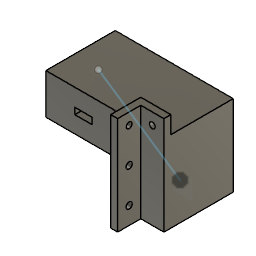
motor_support_strud_Right_v1 (Autodesk Fusion 360 design; units mm, degrees)
part number: 2025-12-05-13-27-42-800
Autodesk Fusion 360 part; units mm, degrees
note: some values were not read from the file. Set by a fixed rule: which sketch regions a step uses.
sketch "Sketch3" plane through (0, 0, 0) normal (0, 0, 1) x (1, 0, 0)
  line L0 (0, 0) -> (-40, 0)
  line L1 (-40, 0) -> (-40, 60)
  line L2 (-40, 60) -> (0, 60)
  line L3 (0, 60) -> (0, 0)
  line L4 (-17.9857, 0) -> (-23.9857, 0)
  line L5 (-23.9857, 0) -> (-23.9857, -20)
  line L6 (-23.9857, -20) -> (-17.9857, -20)
  line L7 (-17.9857, -20) -> (-17.9857, 0)
  line L8 (-40, 0) -> (-23.9857, -20)
  line L9 (-17.9857, 0) -> (2.0143, 0)
  line L10 (2.0143, 0) -> (2.0143, 1.9843)
  line L11 (2.0143, 1.9843) -> (2.0143, 60)
  line L12 (2.0143, 60) -> (0, 60)
  dimension "d16" = 60
  dimension "d17" = 40
  dimension "d18" = 20
  dimension "d19" = 6
  dimension "d63" = 20
  constraint horizontal L0
  constraint vertical L1
  constraint horizontal L2
  constraint vertical L3
  constraint coincident L0.start L3.end
  constraint horizontal L4
  constraint vertical L5
  constraint horizontal L6
  constraint vertical L7
  constraint coincident L0 L4.start
  constraint perpendicular L3 L9
  constraint perpendicular L9 L10
  constraint perpendicular L9 L11
  constraint perpendicular L3 L12
  measures "d16" distance of L0.start L2.end
  measures "d17" distance of L0.start L0.end
  measures "d18" distance of L4.end L5.end
  measures "d19" distance of L5.end L6.end
  measures "d63" distance of L4.start L9.end
extrude "Extrude1" add sketch "Sketch3" along normal blind 85 contours L0 L1 L2 L3 L4 L9 | L0 L4 L5 L6 L7 | L0 L5 L8
sketch "Sketch5" plane through (0, 0, 85) normal (0, 0, 1) x (-1, 0, 0)
  line L0 (23.9857, 20) -> (17.9857, 20)
  line L1 (17.9857, 20) -> (17.9857, 0)
  line L2 (17.9857, 0) -> (0, 0)
  line L3 (0, 0) -> (0, -60)
  line L4 (0, -60) -> (40, -60)
  line L5 (40, -60) -> (40, 0)
  line L6 (40, -60) -> (0, -60)
  line L7 (0, -6) -> (23.9857, -6)
  line L8 (23.9857, -6) -> (23.9857, 0)
  line L9 (40, 0) -> (23.9857, 20)
  line L10 (23.9857, 0) -> (23.9857, 20)
  dimension "d20" = 6
  constraint coincident L4.end L5.start
  constraint coincident L3.end L4.start
  constraint coincident L3 L7.start
  constraint perpendicular L3 L7
  constraint perpendicular L7 L8
  constraint coincident L0.start L9.end
  constraint perpendicular L0 L10
  measures "d20" distance of L2 L7
extrude "Extrude2" cut sketch "Sketch5" against normal blind 15 contours L3 L4 L5 L6 L7 L8 L9 L10
sketch "Sketch6" plane through (-40, 0, 0) normal (-1, 0, 0) x (0, -1, 0)
  line L0 (0, 70) -> (-60, 70)
  line L1 (-60, 70) -> (-60, 0)
  line L2 (-60, 0) -> (0, 0)
  line L3 (-55, 0) -> (-10, 0)
  line L4 (-10, 0) -> (-10, 60)
  line L5 (-10, 60) -> (-55, 60)
  line L6 (-55, 60) -> (-55, 0)
  line L7 (0, 0) -> (0, 70)
  dimension "d23" = 45
  dimension "d27" = 10
  dimension "d28" = 60
  constraint horizontal L3
  constraint vertical L4
  constraint horizontal L5
  constraint vertical L6
  constraint coincident L2 L3.start
  measures "d23" distance of L4.end L5.end
  measures "d27" distance of L4 L7
  measures "d28" distance of L3.start L5.end
extrude "Extrude3" cut sketch "Sketch6" against normal blind 30 contours L2 L3 L4 L5 L6
sketch "Sketch7" plane through (0, 60, 0) normal (0, 1, 0) x (-1, 0, 0)
  line L0 (40, 70) -> (0, 70)
  line L1 (0, 70) -> (0, 0)
  line L2 (0, 0) -> (40, 0)
  line L3 (40, 0) -> (40, 70)
  line L4 (20, 70) -> (20, 10) construction
  circle A0 centre (20, 10) radius 2
  point P0 (20, 10)
  dimension "d29" = 60
  dimension "d30" = 20
  dimension "d31" = 4
  constraint coincident L0 L4.start
  constraint perpendicular L2 L4
  constraint coincident P0 L4.end
  measures "d29" distance of L4.start P0
  measures "d30" distance of L1 L4
  measures "d31" diameter of A0
extrude "Extrude4" cut sketch "Sketch7" against normal blind 57 contours A0
sketch "Sketch8" plane through (0, 55, 0) normal (0, -1, 0) x (1, 0, 0)
  circle A0 centre (-20, 10) radius 2
  line L0 (-40, 60) -> (-40, 0)
  line L1 (-40, 0) -> (-10, 0)
  line L2 (-10, 0) -> (-10, 60)
  line L3 (-10, 60) -> (-40, 60)
  line L4 (-10, 0) -> (-25, 0)
  line L5 (-25, 0) -> (-25, 10)
  line L6 (-20, 15) -> (-10, 15)
  line L7 (-10, 15) -> (-10, 0)
  arc A1 (-20, 15) -> (-25, 10) centre (-20, 10) ccw
  dimension "d34" = 5
  constraint horizontal L4
  constraint vertical L5
  constraint horizontal L6
  constraint vertical L7
  constraint coincident L1.end L2.start
  constraint tangent L5 A1
  constraint tangent L6 A1
  measures "d34" radius of A1
extrude "Extrude5" add sketch "Sketch8" along normal blind 19 contours L1 L2 L4 L5 L6 L7 A1
sketch "Sketch10" plane through (0, 36, 0) normal (0, -1, 0) x (1, 0, 0)
  circle A0 centre (-20, 10) radius 2
  line L0 (-10, 15) -> (-20, 15)
  arc A1 (-20, 15) -> (-25, 10) centre (-20, 10) ccw
  line L1 (-25, 10) -> (-25, 0)
  line L2 (-25, 0) -> (-10, 0)
  line L3 (-10, 0) -> (-10, 15)
  line L4 (-20, 10) -> (-90.5618, 57.3923)
  dimension "d39" = 85
  constraint coincident A0.centre A1.centre
  measures "d39" distance of A0.centre L4.end
sketch "Sketch11" plane through (-40, 0, 0) normal (-1, 0, 0) x (0, -1, 0)
  line L0 (-55, 0) -> (-55, 60)
  line L1 (-55, 60) -> (-10, 60)
  line L2 (-10, 60) -> (-10, 0)
  line L3 (-10, 0) -> (0, 0)
  line L4 (0, 0) -> (0, 70)
  line L5 (0, 70) -> (-60, 70)
  line L6 (-60, 70) -> (-60, 0)
  line L7 (-60, 0) -> (-55, 0)
  line L8 (0, 70) -> (-60, 70)
  line L9 (-60, 35) -> (-55, 35)
  line L10 (-55, 60) -> (-10, 60)
  line L11 (-10, 35) -> (0, 35)
  constraint coincident L4.end L5.start
  constraint coincident L5.end L6.start
  constraint midpoint L6 L9.start
  constraint coincident L0 L9.end
  constraint perpendicular L0 L9
  constraint coincident L0.end L1.start
  constraint coincident L1.end L2.start
  constraint coincident L2 L11.start
  constraint midpoint L4 L11.end
  constraint perpendicular L4 L11
extrude "Extrude6" add sketch "Sketch11" along normal blind 60 contours L0 L1 L2 L4 L5 L6 L8 L9 L10 L11
sketch "Sketch12" plane through (0, 0, 60) normal (0, 0, -1) x (1, 0, 0)
  line L0 (-100, -55) -> (-10, -55)
  line L1 (-10, -55) -> (-10, -10)
  line L2 (-10, -10) -> (-100, -10)
  line L3 (-100, -10) -> (-100, -55)
  line L4 (-94.2104, -42.6) -> (-87.4104, -42.6)
  line L5 (-87.4104, -42.6) -> (-87.4104, -47)
  line L6 (-87.4104, -47) -> (-94.2104, -47)
  line L7 (-94.2104, -47) -> (-94.2104, -42.6)
  dimension "d71" = 6.8
  dimension "d72" = 4.4
  dimension "d73" = 8
  constraint horizontal L4
  constraint vertical L5
  constraint horizontal L6
  constraint vertical L7
  measures "d71" distance of L4.start L4.end
  measures "d72" distance of L4.start L6.end
  measures "d73" distance of L0 L6
extrude "Extrude7" add sketch "Sketch12" along normal blind 5 contours L4 L5 L6 L7
sketch "Sketch13" plane through (-94.2104, 0, 0) normal (-1, 0, 0) x (0, -1, 0)
  line L0 (-42.6, 60) -> (-47, 60)
  line L1 (-47, 60) -> (-47, 55)
  line L2 (-47, 55) -> (-42.6, 55)
  line L3 (-42.6, 55) -> (-42.6, 60)
  line L4 (-47, 58.2513) -> (-42.6, 58.2513)
  line L5 (-42.6, 58.2513) -> (-42.6, 56.9215)
  line L6 (-42.6, 56.9215) -> (-47, 56.9215)
  line L7 (-47, 56.9215) -> (-47, 58.2513)
  constraint horizontal L4
  constraint vertical L5
  constraint horizontal L6
  constraint vertical L7
  constraint coincident L3 L5.end
  constraint coincident L1 L4.start
extrude "Extrude8" cut sketch "Sketch13" against normal blind 2.5 contours L1 L3 L4 L5 L6 L7
sketch "Sketch14" plane through (0, 6, 0) normal (0, 1, 0) x (-1, 0, 0)
  line L0 (23.9857, 85) -> (0, 85)
  line L1 (0, 85) -> (0, 70) construction
  line L2 (0, 70) -> (23.9857, 70)
  line L3 (23.9857, 70) -> (23.9857, 85)
  line L4 (-2.0143, 85) -> (17.9857, 85) construction
  line L5 (17.9857, 85) -> (17.9857, 65) construction
  line L6 (17.9857, 65) -> (-2.0143, 65) construction
  line L7 (-2.0143, 65) -> (-2.0143, 85) construction
  line L8 (17.9857, 85) -> (-2.0143, 65) construction
  line L9 (-2.0143, 85) -> (17.9857, 65) construction
  point P0 (7.9857, 75)
  dimension "d68" = 6
  dimension "d69" = 20
  dimension "d70" = 20
  constraint horizontal L4
  constraint vertical L5
  constraint horizontal L6
  constraint vertical L7
  constraint midpoint P0 L9
  measures "d68" distance of L3 L5
  measures "d69" distance of L4.start L4.end
  measures "d70" distance of L4.start L6.end
hole "Hole3" at (-7.9857, 6, 75) direction (0, -1, 0) diameter 5 depth 10 tip angle 118
sketch "Sketch15" plane through (-23.9857, 0, 0) normal (-1, 0, 0) x (0, -1, 0)
  line L0 (20, 85) -> (-6, 85) construction
  line L1 (-6, 85) -> (-6, 70)
  line L2 (-6, 70) -> (20, 70) construction
  line L3 (20, 70) -> (20, 85) construction
  line L4 (20, 85) -> (0, 85) construction
  line L5 (0, 85) -> (0, 65) construction
  line L6 (0, 65) -> (20, 65) construction
  line L7 (20, 65) -> (20, 85) construction
  line L8 (20, 85) -> (0, 65) construction
  line L9 (0, 85) -> (20, 65) construction
  point P0 (10, 75)
  dimension "d51" = 20
  dimension "d52" = 20
  constraint horizontal L4
  constraint vertical L5
  constraint horizontal L6
  constraint vertical L7
  constraint coincident L0.start L3.end
  constraint midpoint L8 P0
  measures "d51" distance of L0.start L4.end
  measures "d52" distance of L0.start L6.end
hole "Hole4" at (-23.9857, -10, 75) direction (1, 0, 0) diameter 5 depth 6 tip angle 118
sketch "Sketch16" plane through (-40, 0, 0) normal (-1, 0, 0) x (0, -1, 0)
  line L0 (0, 35) -> (-10, 35)
  line L1 (-10, 35) -> (-10, 0)
  line L2 (-10, 0) -> (0, 0)
  line L3 (0, 0) -> (0, 35)
  line L4 (10, 75) -> (10, 0) construction
  point P0 (10, 15)
  point P1 (10, 45)
  constraint vertical L4
  constraint coincident L4 P0
  constraint coincident L4 P1
hole "Hole5" at (-40, -10, 15) at (-40, -10, 45) direction (1, 0, 0) diameter 5.4 depth 25 tip angle 180 counterbore diameter 8.5 counterbore depth 15
extrude "Extrude9" add 1 faces at (0, 22, 23.3333) along direction (1, 0, 0) blind 2.014
sketch "Sketch18" plane through (0, 10, 0) normal (0, 1, 0) x (-1, 0, 0)
  circle A0 centre (20, 10) radius 2
  line L0 (100, 60) -> (10, 60)
  line L1 (10, 60) -> (10, 0)
  line L2 (10, 0) -> (40, 0)
  line L3 (40, 0) -> (40, 35)
  line L4 (40, 35) -> (100, 35)
  line L5 (100, 35) -> (100, 60)
  line L6 (10, 0) -> (25, 0)
  line L7 (25, 0) -> (25, 10)
  line L8 (20, 15) -> (10, 15)
  line L9 (10, 15) -> (10, 0)
  arc A1 (25, 10) -> (20, 15) centre (20, 10) ccw
  dimension "d74" = 5
  constraint horizontal L6
  constraint vertical L7
  constraint horizontal L8
  constraint vertical L9
  constraint coincident L1.end L2.start
  constraint tangent L7 A1
  constraint tangent L8 A1
  measures "d74" radius of A1
extrude "Extrude10" add sketch "Sketch18" along normal blind 3 contours L1 L2 L6 L7 L8 L9 A1
sketch "Sketch19" plane through (0, 0, 0) normal (0, -1, 0) x (1, 0, 0)
  line L0 (-40, 35) -> (-40, 70)
  line L1 (-40, 70) -> (-100, 70)
  line L2 (-100, 70) -> (-100, 35)
  line L3 (-100, 35) -> (-40, 35)
  line L4 (-75, 55) -> (-60, 55)
  line L5 (-60, 55) -> (-60, 49.5)
  line L6 (-60, 49.5) -> (-75, 49.5)
  line L7 (-75, 49.5) -> (-75, 55)
  dimension "d77" = 15
  dimension "d78" = 5.5
  constraint horizontal L4
  constraint vertical L5
  constraint horizontal L6
  constraint vertical L7
  measures "d77" distance of L4.start L4.end
  measures "d78" distance of L4.end L5.end
extrude "Extrude11" cut sketch "Sketch19" against normal blind 10 contours L4 L5 L6 L7
equation "d65 = 20 mm - 17.986 mm"
